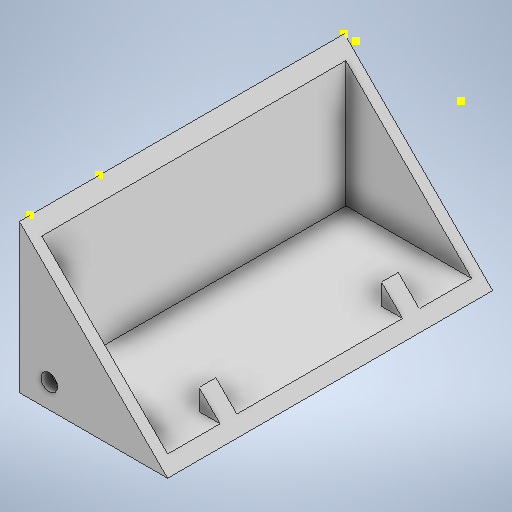
# Autodesk Inventor part: manuDisplayHolder
Saved by Autodesk Inventor 2025 (Build 290162000, 162)
## iProperties
Created: 2024-04-01
Part Number: manuDisplayHolder
Material: Generic
Document SubType Name: Modeling
Designer: 48791
Density: 1 g/cm^3
Appearance: Default
Author: 48791
Autodesk Inventor part; units mm, degrees
ref_plane "YZ Plane" through (0, 0, 0) normal (1, 0, 0) x (0, 1, 0)
ref_plane "XZ Plane" through (0, 0, 0) normal (0, 1, 0) x (-1, 0, 0)
ref_plane "XY Plane" through (0, 0, 0) normal (0, 0, 1) x (1, 0, 0)
sketch "Sketch1" plane through (0, 0, 0) normal (0, 0, 1) x (1, 0, 0)
  line L0 (0, 0) -> (0, -70.71)
  line L1 (0, -70.71) -> (70.71, -70.71)
  line L2 (70.71, -70.71) -> (0, 0)
  dimension "d0" = 70.71
  dimension "d1" = 70.71
  constraints: 6 end point, 1 perpendicular, 1 vertical
  measures "d0" distance of L0.start L0.end
  measures "d1" distance of L0.end L1.end
extrude "Extrusion1" add sketch "Sketch1" along normal blind 155
sketch "Sketch2" plane through (0, -70.71, 0) normal (0, -1, 0) x (1, 0, 0)
  point P0 (0, 0)
sketch "Sketch3" plane through (0, -70.71, 0) normal (0, -1, 0) x (1, 0, 0)
  point P0 (0, 0)
sketch "Sketch4" plane through (0, -70.71, 0) normal (0, -1, 0) x (1, 0, 0)
  point P0 (0, 0)
sketch "Sketch5" plane through (0, -70.71, 0) normal (0, -1, 0) x (1, 0, 0)
  line L0 (65.71, 150) -> (5.71, 150)
  line L1 (5.71, 150) -> (5.71, 5)
  line L2 (5.71, 5) -> (65.71, 5)
  line L3 (65.71, 5) -> (65.71, 150)
  line L4 (70.71, 0) -> (70.71, 155) projected
  line L5 (0, 0) -> (70.71, 0) projected
  dimension "d4" = 60
  dimension "d5" = 145
  dimension "d6" = 5
  dimension "d7" = 5
  constraints: 8 end point, 2 parallel, 1 horizontal, 1 perpendicular
  measures "d4" distance of L2.end L1.end
  measures "d5" distance of L1.end L0.end
  measures "d6" distance between parallel lines of L4 L3
  measures "d7" distance between parallel lines of L5 L2
extrude "Extrusion2" cut sketch "Sketch5" against normal blind 155
sketch "Sketch6" plane through (5.71, -70.71, 150) normal (1, 0, 0) x (0, 0, -1)
  line L0 (0, 0) -> (145, 0)
  line L1 (145, 0) -> (145, 5)
  line L2 (145, 5) -> (0, 5)
  line L3 (0, 5) -> (0, 0)
  point P0 (150, 70.71)
  dimension "d10" = 145
  dimension "d11" = 5
  constraints: 8 end point, 2 parallel, 1 horizontal, 1 perpendicular
  measures "d10" distance of L2.end L1.end
  measures "d11" distance of L1.end L0.end
extrude "Extrusion3" add sketch "Sketch6" along normal blind 60
sketch "Sketch7" plane through (5.71, -5.71, 150) normal (1, 0, 0) x (0, 0, -1)
  point P0 (150, 5.71)
sketch "Sketch8" plane through (65.71, -65.71, 150) normal (0, 0, -1) x (-1, 0, 0)
  point P0 (65.71, 65.71)
sketch "Sketch9" plane through (5.71, -65.71, 150) normal (0, 1, 0) x (1, 0, 0)
  point P0 (-5.71, 150)
sketch "Sketch10" plane through (5.71, -65.71, 150) normal (0, 1, 0) x (1, 0, 0)
  line L0 (60, 145) -> (60, 0) projected
  line L1 (60, 25) -> (50, 25)
  line L2 (50, 25) -> (50, 33)
  line L3 (50, 33) -> (60, 33)
  line L4 (60, 33) -> (60, 25)
  line L5 (60, 112) -> (50, 112)
  line L6 (50, 112) -> (50, 120)
  line L7 (50, 120) -> (60, 120)
  line L8 (60, 120) -> (60, 112)
  line L9 (60, 0) -> (0, 0) projected
  line L10 (0, 145) -> (60, 145) projected
  point P0 (-5.71, 150)
  point P1 (55, 25)
  point P2 (55, 120)
  point P3 (60, 33)
  dimension "d14" = 10
  dimension "d15" = 8
  dimension "d16" = 10
  dimension "d17" = 8
  dimension "d18" = 25
  dimension "d19" = 25
  constraints: 16 end point, 4 parallel, 2 horizontal, 2 midpoint, 2 perpendicular, 2 point on line
  measures "d14" distance of L2.end L3.end
  measures "d15" distance of L1.end L2.end
  measures "d16" distance of L6.end L7.end
  measures "d17" distance of L5.end L6.end
  measures "d18" distance from line of L9 point (55, 25)
  measures "d19" distance from line of L10 point (55, 120)
extrude "Extrusion4" add sketch "Sketch10" along normal blind 10
sketch "Sketch11" plane through (65.71, -65.71, 117) normal (0, 0, -1) x (-1, 0, 0)
  point P0 (65.71, 65.71)
sketch "Sketch12" plane through (65.71, -65.71, 117) normal (0, 0, -1) x (-1, 0, 0)
  line L0 (0, 10) -> (10, 10) projected
  line L1 (0, 0) -> (0, 10)
  line L2 (0, 10) -> (10, 10)
  line L3 (10, 10) -> (0, 0)
  point P0 (65.71, 65.71)
  constraints: 6 end point, 2 perpendicular
extrude "Extrusion5" cut sketch "Sketch12" against normal blind 15
sketch "Sketch13" plane through (65.71, -65.71, 30) normal (0, 0, -1) x (-1, 0, 0)
  line L0 (0, 0) -> (10, 0) projected
  line L1 (0, 0) -> (0, 10) projected
  line L2 (0, 0) -> (0, 10)
  line L3 (10, 0) -> (10, 10) projected
  line L4 (0, 10) -> (10, 10)
  line L5 (10, 10) -> (0, 0)
  point P0 (65.71, 65.71)
  constraints: 6 end point, 1 collinear, 1 perpendicular
extrude "Extrusion6" cut sketch "Sketch13" against normal blind 15 contours L1 L4 L5
sketch "Sketch14" plane through (65.71, -65.71, 150) normal (0, 0, -1) x (-1, 0, 0)
  circle A0 centre (51.4521, 6.4297) radius 4
  point P0 (65.71, 65.71)
  dimension "d26" = 8
  constraints: 1 centre point
  measures "d26" diameter of A0
extrude "Extrusion7" cut sketch "Sketch14" against normal blind 15
sketch "Sketch15" plane through (0, 0, 0) normal (0.7071068, 0.7071068, 0) x (-0.7071068, 0.7071068, 0)
  point P0 (0, 0)
sketch "Sketch16" plane through (0, 0, 0) normal (0.7071068, 0.7071068, 0) x (-0.7071068, 0.7071068, 0)
  point P0 (0, 0)
sketch "Sketch17" plane through (55.71, -65.71, 30) normal (-1, 0, 0) x (0, 0, 1)
  point P0 (-30, 65.71)
sketch "Sketch18" plane through (55.71, -65.71, 30) normal (-1, 0, 0) x (0, 0, 1)
  point P0 (-30, 65.71)
body "Solid1"
